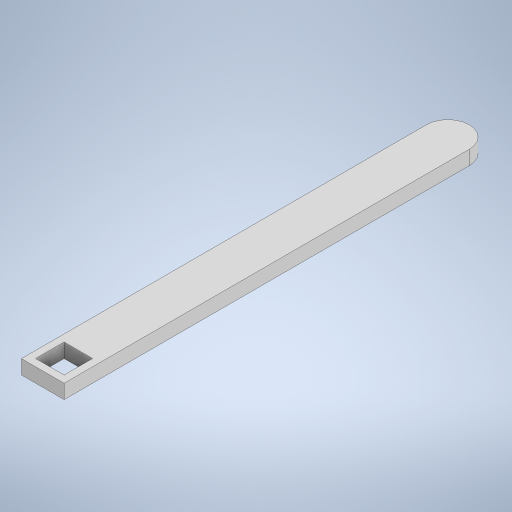
# Autodesk Inventor part: V3_O4
Saved by Autodesk Inventor 2023.1 (Build 271208000, 208)
## iProperties
Created: 2023-04-22
Part Number: V3_O4
Material: Generisch
Document SubType Name: Sheet Metal
Designer: marco
Density: 1 g/cm^3
Sheet Metal Rule: Standard_mm
Appearance: Vorgabe
Author: marco
Autodesk Inventor part; units mm, degrees
ref_plane "YZ Plane" through (0, 0, 0) normal (1, 0, 0) x (0, 1, 0)
ref_plane "XZ Plane" through (0, 0, 0) normal (0, 1, 0) x (-1, 0, 0)
ref_plane "XY Plane" through (0, 0, 0) normal (0, 0, 1) x (1, 0, 0)
sketch "Skizze1" plane through (0, 0, 0) normal (0, 1, 0) x (-1, 0, 0)
  line L0 (0, 0) -> (6, 0)
  line L1 (6, 0) -> (6, -57)
  line L2 (3, -60) -> (3, -60)
  line L3 (0, -57) -> (0, 0)
  arc A0 (3, -60) -> (6, -57) centre (3, -57) ccw
  arc A1 (0, -57) -> (3, -60) centre (3, -57) ccw
  line L4 (1, -1) -> (5, -1)
  line L5 (5, -1) -> (5, -5)
  line L6 (5, -5) -> (1, -5)
  line L7 (1, -5) -> (1, -1)
  point P0 (6, -60)
  point P1 (0, -60)
  point P2 (3, -60)
  dimension "d0" = 6
  dimension "d1" = 60
  dimension "d2" = 3
  dimension "d3" = 4
  dimension "d4" = 4
  constraints: 16 end point, 4 parallel, 4 point on circle, 4 point on line, 4 tangent, 2 centre point, 2 horizontal, 2 perpendicular, 1 concentric
  measures "d0" distance of point (6, -60) point (0, -60)
  measures "d1" distance of L0.end point (6, -60)
  measures "d2" radius of A0
  measures "d3" distance of L5.end L6.end
  measures "d4" distance of L4.end L5.end
extrude "Extrusion1" add sketch "Skizze1" along normal blind 2
equation "\"Biegeradius\" = Stärke"
equation "\"BreiteBiegungsfreistellung\" = Stärke"
equation "\"TiefeBiegungsfreistellung\" = 0.5 * Stärke"
equation "\"GrößeEckenfreistellung\" = 4 * Stärke"
equation "\"MinimalRest\" = 2 * Stärke"
equation "\"Übergangsradius\" = Biegeradius"
equation "\"JacobiRadiusGröße\" = Biegeradius"
equation "\"Abstandsgröße\" = Stärke"
equation "\"Stärke\" = 0.5"
